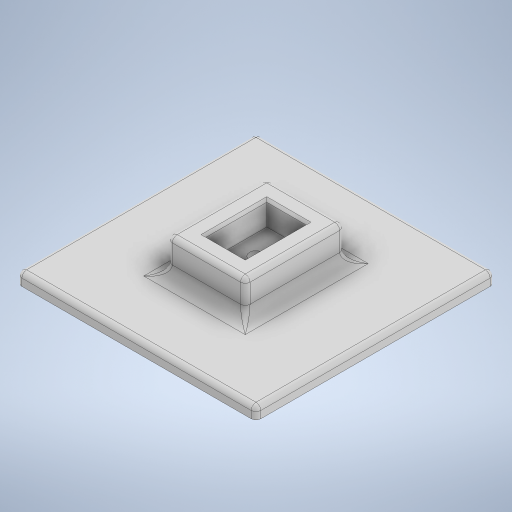
# Autodesk Inventor part: base_frame
Saved by Autodesk Inventor 2023 (Build 270158000, 158)
## iProperties
Created: 2023-11-15
Part Number: base_frame
Material: Generic
Document SubType Name: Modeling
Designer: zavrel
Density: 1 g/cm^3
Appearance: Default
Author: zavrel
Autodesk Inventor part; units mm, degrees
ref_plane "YZ Plane" through (0, 0, 0) normal (1, 0, 0) x (0, 1, 0)
ref_plane "XZ Plane" through (0, 0, 0) normal (0, 1, 0) x (-1, 0, 0)
ref_plane "XY Plane" through (0, 0, 0) normal (0, 0, 1) x (1, 0, 0)
sketch "Sketch1" plane through (0, 0, 0) normal (0, 1, 0) x (-1, 0, 0)
  line L0 (0, 0) -> (100, 0)
  line L1 (100, 0) -> (100, -100)
  line L2 (100, -100) -> (0, -100)
  line L3 (0, -100) -> (0, 0)
  dimension "d0" = 100
  dimension "d1" = 100
  constraints: 8 end point, 2 parallel, 1 horizontal, 1 perpendicular
  measures "d0" distance of L2.end L0.start
  measures "d1" distance of L0.start L0.end
extrude "Extrusion1" add sketch "Sketch1" along normal blind 5
sketch "Sketch2" plane through (0, 5, 0) normal (0, 1, 0) x (1, 0, 0)
  line L0 (0, 100) -> (-100, 100) projected
  line L1 (-100, 100) -> (-100, 0) projected
  line L2 (-100, 0) -> (0, 0) projected
  line L3 (0, 0) -> (0, 100) projected
  line L4 (-58.25, 37.25) -> (-41.75, 37.25)
  line L5 (-41.75, 37.25) -> (-41.75, 62.75)
  line L6 (-41.75, 62.75) -> (-58.25, 62.75)
  line L7 (-58.25, 62.75) -> (-58.25, 37.25)
  line L8 (-66.25, 29.25) -> (-33.75, 29.25)
  line L9 (-33.75, 29.25) -> (-33.75, 70.75)
  line L10 (-33.75, 70.75) -> (-66.25, 70.75)
  line L11 (-66.25, 70.75) -> (-66.25, 29.25)
  line L12 (-100, 100) -> (-100, 0) construction
  line L13 (0, 100) -> (-100, 100) construction
  line L14 (-100, 0) -> (0, 100) construction
  line L15 (0, 100) -> (-100, 100) construction
  line L16 (-100, 100) -> (0, 0) construction
  line L17 (-66.25, 29.25) -> (-33.75, 70.75) construction
  line L18 (-66.25, 70.75) -> (-33.75, 29.25) construction
  point P0 (-50, 50)
  dimension "d7" = 16.5
  dimension "d8" = 25.5
  dimension "d10" = 8
  constraints: 26 end point, 5 equal length, 3 perpendicular, 2 midpoint, 1 horizontal, 3 other
  measures "d7" distance of L5.end L6.end
  measures "d8" distance of L6.end L4.start
  measures "d10" distance between parallel lines of L7 L11
extrude "Extrusion2" add sketch "Sketch2" along normal blind 15 contours L11 L10 L9 L8
sketch "Sketch3" plane through (0, 5, 0) normal (0, 1, 0) x (1, 0, 0)
  line L0 (-58.25, 37.25) -> (-41.75, 37.25) projected
  line L1 (-41.75, 37.25) -> (-41.75, 62.75) projected
  line L2 (-41.75, 62.75) -> (-58.25, 62.75) projected
  line L3 (-58.25, 62.75) -> (-58.25, 37.25) projected
  point P0 (0, 0)
extrude "Extrusion3" add sketch "Sketch3" along normal blind 5
sketch "Sketch4" plane through (0, 10, 0) normal (0, 1, 0) x (1, 0, 0)
  line L0 (-41.75, 62.75) -> (-41.75, 37.25) projected
  line L1 (-58.25, 62.75) -> (-41.75, 62.75) projected
  line L2 (-58.25, 37.25) -> (-58.25, 62.75) projected
  line L3 (-41.75, 37.25) -> (-58.25, 37.25) projected
  line L4 (-58.25, 37.25) -> (-41.75, 62.75) construction
  line L5 (-58.25, 62.75) -> (-41.75, 37.25) construction
  circle A0 centre (-50, 50) radius 2.75
  point P0 (0, 0)
  dimension "d15" = 5.5
  constraints: 4 end point, 1 centre point, 1 midpoint
  measures "d15" diameter of A0
extrude "Extrusion4" cut sketch "Sketch4" against normal through all contours A0
sketch "Sketch5" plane through (0, 0, 0) normal (0, -1, 0) x (1, 0, 0)
  circle A0 centre (-50, -50) radius 2.75 projected
  line L0 (0, -100) -> (-100, -100) projected
  line L1 (0, 0) -> (0, -100) projected
  line L2 (-100, 0) -> (0, 0) projected
  line L3 (-100, -100) -> (-100, 0) projected
  circle A1 centre (-50, -50) radius 4.5
  dimension "d18" = 9
  constraints: 1 centre point, 1 coincident
  measures "d18" diameter of A1
extrude "Extrusion5" cut sketch "Sketch5" against normal blind 5.5 contours A0 | A1
fillet "Fillet1" radius 5 4 edges at (-66.25, 5, -50) (-50, 5, -70.75) (-50, 5, -29.25) (-33.75, 5, -50)
fillet "Fillet2" radius 2 20 edges at (-33.75, 20, -50) (-50, 20, -70.75) (-66.25, 20, -50) (-50, 20, -29.25) (-67.7145, 6.4645, -27.7855) (-66.25, 15, -29.25) (-67.7145, 6.4645, -72.2145) (-66.25, 15, -70.75) (-32.2855, 6.4645, -27.7855) (-33.75, 15, -29.25) (-32.2855, 6.4645, -72.2145) (-33.75, 15, -70.75) (0, 5, -50) (-50, 5, 0) (0, 2.5, 0) (-50, 5, -100) (0, 2.5, -100) (-100, 2.5, -100) (-100, 5, -50) (-100, 2.5, 0)
chamfer "Chamfer1" distance 1 angle 45 4 edges at (-58.25, 20, -50) (-50, 20, -62.75) (-50, 20, -37.25) (-41.75, 20, -50)
body "Solid1"
